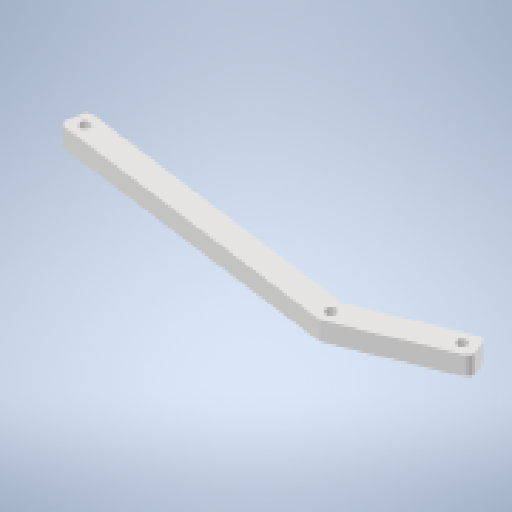
# Autodesk Inventor part: Part2
Saved by Autodesk Inventor 2023 (Build 270158000, 158)
## iProperties
Created: 2023-03-01
Part Number: Part2
Material: Generic
Document SubType Name: Modeling
Designer: Gabriel - T3 CAD
Density: 1 g/cm^3
Appearance: Default
Author: Gabriel - T3 CAD
Autodesk Inventor part; units mm, degrees
ref_plane "YZ Plane" through (0, 0, 0) normal (1, 0, 0) x (0, 1, 0)
ref_plane "XZ Plane" through (0, 0, 0) normal (0, 1, 0) x (-1, 0, 0)
ref_plane "XY Plane" through (0, 0, 0) normal (0, 0, 1) x (1, 0, 0)
sketch "Sketch1" plane through (0, 0, 0) normal (0, 1, 0) x (-1, 0, 0)
  line L0 (0, 0) -> (190.5, 0)
  line L1 (190.5, 0) -> (47.0141, 19.3142)
  line L2 (47.0141, 19.3142) -> (0, 0)
  line L3 (2.413, -5.8737) -> (-2.413, 5.8737)
  line L4 (-2.413, 5.8737) -> (45.388, 25.5111)
  line L5 (47.0663, 12.4707) -> (2.413, -5.8737)
  line L6 (41.2492, 26.4974) -> (39.555, 13.9109)
  line L7 (48.6964, 12.6805) -> (189.6529, -6.2932)
  line L8 (189.6529, -6.2932) -> (191.3471, 6.2932)
  line L9 (191.3471, 6.2932) -> (47.0181, 25.7209)
  arc A0 (47.0181, 25.7209) -> (45.388, 25.5111) centre (46.5945, 22.5743) ccw
  arc A1 (48.6964, 12.6805) -> (47.0663, 12.4707) centre (48.2728, 9.5338) ccw
  circle A2 centre (47.0141, 19.3142) radius 2.5797
  circle A3 centre (190.5, 0) radius 2.5797
  circle A4 centre (0, 0) radius 2.5797
  line L10 (191.3471, 6.2932) -> (189.6529, -6.2932)
  line L11 (189.6529, -6.2932) -> (192.7995, -6.7168)
  line L12 (196.3697, -3.9937) -> (197.2168, 2.2995)
  line L13 (194.4937, 5.8697) -> (191.3471, 6.2932)
  arc A5 (197.2168, 2.2995) -> (194.4937, 5.8697) centre (194.0702, 2.7231) ccw
  arc A6 (192.7995, -6.7168) -> (196.3697, -3.9937) centre (193.2231, -3.5702) ccw
  line L14 (-2.413, 5.8737) -> (2.413, -5.8737)
  line L15 (2.413, -5.8737) -> (-0.5238, -7.0802)
  line L16 (-4.6672, -5.3498) -> (-7.0802, 0.5238)
  line L17 (-5.3498, 4.6672) -> (-2.413, 5.8737)
  arc A7 (-5.3498, 4.6672) -> (-7.0802, 0.5238) centre (-4.1433, 1.7303) ccw
  arc A8 (-4.6672, -5.3498) -> (-0.5238, -7.0802) centre (-1.7303, -4.1433) ccw
  point P0 (195.9461, -7.1404)
  point P1 (-3.4607, -8.2867)
  dimension "d0" = 190.5
  dimension "d1" = 150
  dimension "d2" = 12.7
  dimension "d3" = 3.175
  dimension "d4" = 5.1594
  dimension "d6" = 6.35
  dimension "d7" = 3.175
  dimension "d8" = 6.35
  dimension "d9" = 3.175
  dimension "d12" = 144.78
  constraints: 36 end point, 12 point on circle, 12 tangent, 9 centre point, 9 parallel, 6 point on line, 5 equal radius, 5 perpendicular, 3 coincident, 2 midpoint, 1 collinear, 1 equal length, 1 horizontal
  measures "d0" distance of L0.end L0.start
  measures "d1" angle of L2 L1
  measures "d2" distance of L3.start L3.end
  measures "d3" radius of A0
  measures "d4" diameter of A2
  measures "d6" distance of L7.end point (195.946, -7.14)
  measures "d7" radius of A5
  measures "d8" distance of L3.start point (-3.461, -8.287)
  measures "d9" radius of A7
  measures "d12" distance of L0.end L1.end
extrude "Extrusion1" add sketch "Sketch1" along normal blind 9.525 contours A4 L2 A2 L1 A3 L0 L7 A1 L5 | L0 L5 L3 A4 | A4 L3 L4 L6 L2 | L3 L15 A8 L16 A7 L17 A4 | L6 L4 A0 L9 L8 A3 L1 A2 L2 | L0 A3 L8 L7 | L8 A3 L13 A5 L12 A6 L11
body "Solid1"
